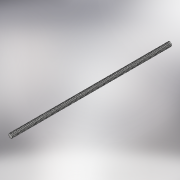
# Autodesk Inventor part: TR8x8 lead screw
Saved by Autodesk Inventor 2020 (Build 240168000, 168)
## iProperties
Created: 2018-04-20
Part Number: TR8x8 lead screw
Material: Generic
Document SubType Name: Modeling
Designer: PC  USER
Density: 1 g/cm^3
Appearance: Default
Author: PC  USER
Autodesk Inventor part; units mm, degrees
ref_plane "YZ Plane" through (0, 0, 0) normal (1, 0, 0) x (0, 1, 0)
ref_plane "XZ Plane" through (0, 0, 0) normal (0, 1, 0) x (-1, 0, 0)
ref_plane "XY Plane" through (0, 0, 0) normal (0, 0, 1) x (1, 0, 0)
sketch "Sketch1" plane through (0, 0, 0) normal (0, 1, 0) x (-1, 0, 0)
  circle A0 centre (0, 0) radius 3.5
  dimension "d0" = 7
  constraints: 1 centre point, 1 coincident
  measures "d0" diameter of A0
extrude "Extrusion1" add sketch "Sketch1" along normal mid plane 300
sketch "Sketch3" plane through (0, 0, 0) normal (1, 0, 0) x (0, 1, 0)
  line L0 (-150, 3.5) -> (-150, -3.5) projected
  line L1 (150, -3.5) -> (150, 3.5) projected
  line L2 (150, 3.5) -> (149, 3.5)
  line L3 (149, 3.5) -> (149, 4)
  line L4 (149, 4) -> (150, 4)
  line L5 (150, 4) -> (150, 3.5)
  line L6 (-199.5, 0) -> (199.5, 0) projected
  point P0 (0, 0)
  dimension "d7" = 1
  dimension "d8" = 0
  dimension "d9" = 3.5
  dimension "d10" = 0.5
  constraints: 8 end point, 2 parallel, 1 horizontal, 1 perpendicular
  measures "d7" distance of L3.end L4.end
  measures "d8" distance between parallel lines of L1 L5
  measures "d9" distance between parallel lines of L6 L2
  measures "d10" distance of L2.end L3.end
coil "Coil1" sketch "Sketch3" operation add axis through (0, -10, 0) along (0, -1, 0) pitch 2 turns 150 hand right
body "Solid1"
